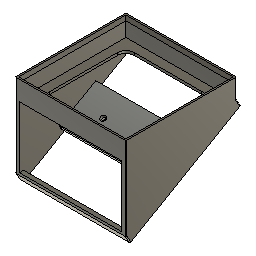
PanaThermoMount_V3 (Autodesk Fusion 360 design; units mm, degrees)
part number: 2025-11-10-19-08-12-267
Autodesk Fusion 360 part; units mm, degrees
sketch "BasePlate" plane through (0, 0, 0) normal (0, 0, 1) x (1, 0, 0)
  line L0 (64.5, 65.5) -> (-64.5, 65.5)
  line L1 (-65.5, 64.5) -> (-65.5, -64.5)
  line L2 (-64.5, -65.5) -> (64.5, -65.5)
  line L3 (65.5, -64.5) -> (65.5, 64.5)
  line L4 (65.5, 65.5) -> (-65.5, -65.5) construction
  line L5 (-65.5, 65.5) -> (65.5, -65.5) construction
  line L6 (60.5, 60.5) -> (-60.5, 60.5)
  line L7 (-60.5, 60.5) -> (-60.5, -60.5)
  line L8 (-60.5, -60.5) -> (60.5, -60.5)
  line L9 (60.5, -60.5) -> (60.5, 60.5)
  line L10 (60.5, 60.5) -> (-60.5, -60.5) construction
  line L11 (-60.5, 60.5) -> (60.5, -60.5) construction
  line L12 (40, 50) -> (-40, 50)
  line L13 (-50, 40) -> (-50, -40)
  line L14 (-40, -50) -> (40, -50)
  line L15 (50, -40) -> (50, 40)
  line L16 (50, 50) -> (-50, -50) construction
  line L17 (-50, 50) -> (50, -50) construction
  arc A0 (-64.5, 65.5) -> (-65.5, 64.5) centre (-64.5, 64.5) ccw
  arc A1 (65.5, 64.5) -> (64.5, 65.5) centre (64.5, 64.5) ccw
  arc A2 (64.5, -65.5) -> (65.5, -64.5) centre (64.5, -64.5) ccw
  arc A3 (-65.5, -64.5) -> (-64.5, -65.5) centre (-64.5, -64.5) ccw
  arc A4 (-40, 50) -> (-50, 40) centre (-40, 40) ccw
  arc A5 (50, 40) -> (40, 50) centre (40, 40) ccw
  arc A6 (40, -50) -> (50, -40) centre (40, -40) ccw
  arc A7 (-50, -40) -> (-40, -50) centre (-40, -40) ccw
  dimension "d1" = 131
  dimension "d2" = 131
  dimension "d3" = 121
  dimension "d4" = 121
  dimension "d5" = 100
  dimension "d6" = 100
  dimension "d7" = 1
  dimension "d19" = 10
  constraint horizontal L0
  constraint perpendicular L0 L1
  constraint parallel L0 L2
  constraint parallel L1 L3
  constraint coincident L4 origin
  constraint coincident L5 origin
  constraint horizontal L6
  constraint perpendicular L6 L7
  constraint parallel L6 L8
  constraint parallel L7 L9
  constraint coincident L10 origin
  constraint coincident L11 origin
  constraint horizontal L12
  constraint perpendicular L12 L13
  constraint parallel L12 L14
  constraint parallel L13 L15
  constraint coincident L16 origin
  constraint coincident L17 origin
  constraint coincident L5.start L0
  constraint coincident L5.start L1
  constraint tangent L0 A0
  constraint tangent L1 A0
  constraint coincident L4.start L0
  constraint coincident L4.start L3
  constraint tangent L0 A1
  constraint tangent L3 A1
  constraint equal A0 A1
  constraint coincident L5.end L3
  constraint coincident L5.end L2
  constraint tangent L3 A2
  constraint tangent L2 A2
  constraint equal A0 A2
  constraint coincident L4.end L2
  constraint coincident L4.end L1
  constraint tangent L2 A3
  constraint tangent L1 A3
  constraint equal A0 A3
  constraint coincident L17.start L12
  constraint coincident L17.start L13
  constraint tangent L12 A4
  constraint tangent L13 A4
  constraint coincident L16.start L12
  constraint coincident L16.start L15
  constraint tangent L12 A5
  constraint tangent L15 A5
  constraint equal A4 A5
  constraint coincident L17.end L15
  constraint coincident L17.end L14
  constraint tangent L15 A6
  constraint tangent L14 A6
  constraint equal A4 A6
  constraint coincident L16.end L14
  constraint coincident L16.end L13
  constraint tangent L14 A7
  constraint tangent L13 A7
  constraint equal A4 A7
  measures "d1" distance of L4.end L5.end
  measures "d2" distance of L5.start L4.end
  measures "d3" distance of L7.end L8.end
  measures "d4" distance of L6.end L7.end
  measures "d5" distance of L16.end L17.end
  measures "d6" distance of L17.start L16.end
  measures "d7" radius of A0
  measures "d19" radius of A4
extrude "Extrude1" add sketch "BasePlate" along normal blind 23 contours L0 L1 L2 L3 A0 A1 A2 A3 makes body 1
extrude "Extrude2" add sketch "BasePlate" along normal blind 3 contours L6 L7 L8 L9 bodies 1
extrude "Extrude3" add sketch "BasePlate" against normal blind 100 contours L0 L1 L2 L3 A0 A1 A2 A3 bodies 1
chamfer "Chamfer5" distance 3 angle 45 4 edges at (0, -60.5, 23) (60.5, 0, 23) (0, 60.5, 23) (-60.5, 0, 23) on bodies 1
ref_plane "WorkPlane1" through (0, 65.5, 0) normal (0, -0.5, 0.866025) x (-1, 0, 0)
split "Split1" by plane through (0, 65.5, 0) normal (0, -0.5, 0.866025) bodies 1 makes body 2 at (-21.5, -65.5, -9.8776)
delete_body "RemoveBody1" bodies 1
sketch "MountBridge" plane through (0, 16.375, -28.3623) normal (0, 0.5, -0.866025) x (-1, 0, 0)
  line L0 (65.5, -93.3864) -> (65.5, 55.57)
  ellipse E0 centre (64.5, 55.57) end of major axis (64.5, 56.7247) minor radius 1 (65.5, 55.57) -> (64.5, 56.7247) ccw
  line L1 (64.5, 56.7247) -> (-64.5, 56.7247)
  ellipse E1 centre (-64.5, 55.57) end of major axis (-64.5, 56.7247) minor radius 1 (-64.5, 56.7247) -> (-65.5, 55.57) ccw
  line L2 (-65.5, 55.57) -> (-65.5, -93.3864)
  ellipse E2 centre (-64.5, -93.3864) end of major axis (-64.5, -94.5411) minor radius 1 (-65.5, -93.3864) -> (-64.5, -94.5411) ccw
  line L3 (-64.5, -94.5411) -> (64.5, -94.5411)
  ellipse E3 centre (64.5, -93.3864) end of major axis (64.5, -94.5411) minor radius 1 (64.5, -94.5411) -> (65.5, -93.3864) ccw
  line L4 (60.5, -88.7676) -> (-60.5, -88.7676)
  line L5 (-60.5, -88.7676) -> (-60.5, 50.9512)
  line L6 (-60.5, 50.9512) -> (60.5, 50.9512)
  line L7 (60.5, 50.9512) -> (60.5, -88.7676)
  line L8 (-60.5, 9.7957) -> (60.5, 9.7957)
  line L9 (60.5, 9.7957) -> (60.5, -40.2043)
  line L10 (60.5, -40.2043) -> (-60.5, -40.2043)
  line L11 (-60.5, -40.2043) -> (-60.5, 9.7957)
  line L12 (-60.5, 50.9512) -> (-60.5, -88.7676)
  line L13 (-60.5, -88.7676) -> (-60.5, -52.3945)
  line L14 (-60.5, -52.3945) -> (-60.5, 52.3945)
  line L15 (-60.5, 52.3945) -> (-60.5, 50.9512)
  dimension "d29" = 50
  constraint horizontal L8
  constraint vertical L9
  constraint horizontal L10
  constraint vertical L11
  constraint coincident L5 L8.start
  measures "d29" distance of L8.start L10.end
extrude "Extrude7" add sketch "MountBridge" along normal blind 10 bodies 2
extrude "Extrude8" add sketch "MountBridge" along normal blind 5 contours L5 L7 L8 L9 L10 L11 L12 L14 bodies 2
sketch "MountHoles" plane through (0, 16.375, -28.3623) normal (0, 0.5, -0.866025) x (-1, 0, 0)
  circle A0 centre (30, -15.2043) radius 2.5
  circle A1 centre (-30, -15.2043) radius 2.5
  line L0 (-60.5, 9.7957) -> (60.5, 9.7957)
  dimension "d34" = 5
  dimension "d35" = 30
  dimension "d36" = 5
  dimension "d37" = 30
  dimension "d38" = 25
  dimension "d39" = 25
  measures "d34" diameter of A0
  measures "d35" horizontal distance of A0.centre origin
  measures "d36" diameter of A1
  measures "d37" horizontal distance of origin A1.centre
  measures "d38" distance of A0.centre L0
  measures "d39" distance of A1.centre L0
hole "Hole1" at (30, 3.2077, -35.9645) direction (0, 0.5, -0.866025) diameter 3.4 depth 5 tip angle 180 countersink diameter 6.3 countersink angle 90 bodies 2
hole "Hole2" at (-30, 3.2077, -35.9645) direction (0, 0.5, -0.866025) diameter 3.4 depth 5 tip angle 180 countersink diameter 6.3 countersink angle 90 bodies 2
extrude "Extrude9" cut 1 faces at (-20.1667, -60.5, -48.4974) along direction (0, -1, 0) blind 5 on bodies 2 bodies 2
